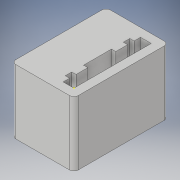
# Autodesk Inventor part: clip_fit_prototype
Saved by Autodesk Inventor 2019 (Build 230136000, 136)
## iProperties
Created: 2019-09-25
Part Number: clip_fit_prototype
Material: Generic
Document SubType Name: Modeling
Designer: Alex
Density: 1 g/cm^3
Appearance: Default
Author: Alex
Autodesk Inventor part; units mm, degrees
ref_plane "YZ Plane" through (0, 0, 0) normal (1, 0, 0) x (0, 1, 0)
ref_plane "XZ Plane" through (0, 0, 0) normal (0, 1, 0) x (-1, 0, 0)
ref_plane "XY Plane" through (0, 0, 0) normal (0, 0, 1) x (1, 0, 0)
sketch "Sketch1" plane through (0, 0, 0) normal (0, 1, 0) x (-1, 0, 0)
  line L0 (0, 0) -> (2.5, 0)
  line L1 (2.5, -18) -> (0, -18)
  line L2 (0, -18) -> (0, 0)
  line L3 (11.5, 2) -> (-1, 2)
  line L4 (-2, 1) -> (-2, -19)
  line L5 (-1, -20) -> (11.5, -20)
  line L6 (12.5, -19) -> (12.5, 1)
  line L7 (2.5, -1.5) -> (3.5, -1.5)
  line L8 (2.5, -16.5) -> (3.5, -16.5)
  line L9 (3.5, -1.5) -> (3.5, -3)
  line L10 (3.5, -3) -> (2.5, -3)
  line L11 (3.5, -16.5) -> (3.5, -15)
  line L12 (3.5, -15) -> (2.5, -15)
  line L13 (2.5, -1.5) -> (2.5, 0)
  line L14 (2.5, -3) -> (2.5, -15)
  line L15 (2.5, -16.5) -> (2.5, -18)
  arc A0 (-1, 2) -> (-2, 1) centre (-1, 1) ccw
  arc A1 (-2, -19) -> (-1, -20) centre (-1, -19) ccw
  arc A2 (11.5, -20) -> (12.5, -19) centre (11.5, -19) ccw
  arc A3 (12.5, 1) -> (11.5, 2) centre (11.5, 1) ccw
  dimension "d0" = 18
  dimension "d1" = 2.5
  dimension "d3" = 2
  dimension "d4" = 2
  dimension "d5" = 2
  dimension "d7" = 1
  dimension "d8" = 15
  dimension "d10" = 1.5
  dimension "d11" = 1.5
  dimension "d12" = 1
  constraints: 32 end point, 8 point on circle, 8 tangent, 4 centre point, 3 equal radius, 3 horizontal, 3 parallel, 2 collinear, 2 vertical, 1 perpendicular, 1 point on line
  measures "d0" distance of L0.end L1.start
  measures "d1" distance of L1.start L1.end
  measures "d3" distance between parallel lines of L4 L2
  measures "d4" distance between parallel lines of L3 L0
  measures "d5" distance between parallel lines of L5 L1
  measures "d7" distance of L7.start L7.end
  measures "d8" distance between parallel lines of L8 L7
  measures "d10" distance of L7.end L9.end
  measures "d11" distance of L8.end L11.end
  measures "d12" radius of A0
sketch "Sketch3" plane through (0, 0, 0) normal (0, 1, 0) x (-1, 0, 0)
  point P0 (0, 0)
extrude "Extrusion1" add sketch "Sketch1" along normal blind 15
sketch "Sketch4" plane through (0, 15, 0) normal (0, 1, 0) x (1, 0, 0)
  point P0 (0, 0)
sketch "Sketch5" plane through (0, 15, 0) normal (0, 1, 0) x (1, 0, 0)
  line L0 (-2.5, 5.75) -> (-3.5, 5.75)
  line L1 (-3.5, 5.75) -> (-3.5, 12.25)
  line L2 (-3.5, 12.25) -> (-2.5, 12.25)
  line L3 (-2.5, 12.25) -> (-2.5, 5.75)
  line L4 (-2.5, 3) -> (-2.5, 15) projected
  line L5 (-11.5, -2) -> (1, -2) projected
  point P0 (0, 0)
  dimension "d15" = 1
  dimension "d16" = 6.5
  dimension "d17" = 0
  dimension "d18" = 7.75
  constraints: 8 end point, 2 parallel, 1 horizontal, 1 perpendicular
  measures "d15" distance between parallel lines of L1 L3
  measures "d16" distance between parallel lines of L2 L0
  measures "d17" distance between parallel lines of L4 L3
  measures "d18" distance between parallel lines of L5 L0
extrude "Extrusion2" cut sketch "Sketch5" against normal blind 13
body "Solid1"
